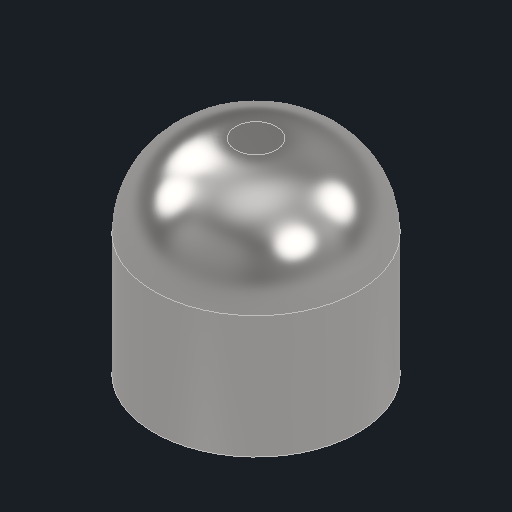
# Autodesk Inventor part: Top Lock Cap
Saved by Autodesk Inventor 2027.1 (Build 311270010, 270A)
## iProperties
Created: 2025-09-16
Material: Brass, Soft Yellow
Document SubType Name: Modeling
Designer: SD
Density: 8.47 g/cm^3
Appearance: Semi-Polished
Mass: 5.28497 g
Surface Area: 4.96433 cm^2
Volume: 0.623963 cm^3
Project: Automatic Tea Steeping mechanism
Part Number: Top Lock Cap
Length: 10.000 mm
BOM-Mass: 0.00490
BOM-Area: 0.000
Diameter: 10.000 mm
Procurement: Fabricate - 1st round
Build Stage: 1
Preferred Material: C36000 Brass
Author: SD
Title: Top Lock Cap
Autodesk Inventor part; units mm, degrees
ref_plane "YZ Plane" through (0, 0, 0) normal (1, 0, 0) x (0, 1, 0)
ref_plane "XZ Plane" through (0, 0, 0) normal (0, 1, 0) x (-1, 0, 0)
ref_plane "XY Plane" through (0, 0, 0) normal (0, 0, 1) x (1, 0, 0)
sketch "Sketch4" plane through (0, 0, 0) normal (0, 1, 0) x (-1, 0, 0)
  circle A0 centre (0, 0) radius 5
  constraints: 1 centre point, 1 coincident, 1 other
extrude "Extrusion2" add sketch "Sketch4" along normal mid plane 10
fillet "Fillet5" radius 4 1 edges at (5, 5, 0)
sketch "Sketch14" plane through (0, -5, 0) normal (0, -1, 0) x (1, 0, 0)
  circle A0 centre (0, 0) radius 1 projected
  constraints: 1 coincident
hole "Hole6" at (0, -5, 0) direction (0, 1, 0) diameter 3 depth 7
sketch "Sketch15" plane through (0, 0, 0) normal (1, 0, 0) x (0, 1, 0)
  line L0 (-5, 5) -> (-5, -5) projected
  point P0 (0, 0)
  point P1 (-1.5, 0)
  dimension "d109" = 3.5
  constraints: 1 horizontal alignment
  measures "d109" distance from line of point (-1.5, 0) L0
hole "Hole7" at (0, -1.5, 0) direction (-1, 0, 0) diameter 2.85 depth 10.4 thread size "M3.5x0.6" class "6H" standard "ISO Metric profile"
body "Solid2"
